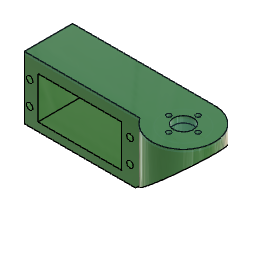
Coxa v8 (Autodesk Fusion 360 design; units mm, degrees)
Autodesk Fusion 360 part; units mm, degrees
sketch "Sketch1" plane through (0, 0, 0) normal (0, 0, 1) x (1, 0, 0)
  circle A0 centre (0, 0) radius 10
  dimension "d1" = 20
  constraint coincident A0.centre origin
  measures "d1" diameter of A0
extrude "Extrude1" add sketch "Sketch1" along normal blind 0.5 makes body 1
sketch "Sketch2" plane through (0, 0, 0) normal (0, 0, -1) x (1, 0, 0)
  circle A0 centre (0, 0) radius 10
  circle A1 centre (0, 0) radius 15
  dimension "d4" = 30
  constraint concentric A0 A1
  measures "d4" diameter of A1
extrude "Extrude2" add sketch "Sketch2" along normal blind 4 separate body makes body 2
sketch "Sketch3" plane through (0, 0, 0) normal (0, 1, 0) x (1, 0, 0)
sketch "Sketch4" plane through (0, 0, 0) normal (0, 1, 0) x (1, 0, 0)
  line L0 (-12.3324, 0) -> (-15, 0)
  line L1 (-12.3324, 3.9554) -> (-12.3324, 0)
  line L2 (-15.0407, 3.9554) -> (-47.0433, 16.0142)
  line L3 (-15, 0) -> (-47.0492, -12.0611)
  line L4 (-15.0407, 3.9554) -> (-12.3324, 3.9554)
  arc A0 (-47.0433, 16.0142) -> (-47.0492, -12.0611) centre (-52.3324, 1.9777) ccw
  dimension "d8" = 30
  constraint horizontal L0
  constraint vertical L1
  constraint tangent L2 A0
  constraint tangent L3 A0
  measures "d8" diameter of A0
extrude "Extrude3" add sketch "Sketch4" along normal mid plane 30 bodies 2
sketch "Sketch5" plane through (0, 0, 0) normal (0, 0, 1) x (1, 0, 0)
  line L0 (-12.2989, -8.5565) -> (-47, -8.5565)
  line L1 (-47, -8.5565) -> (-47, -15)
  line L2 (-47, -15) -> (-12.2989, -15)
  line L3 (-12.2989, -15) -> (-12.2989, -8.5565)
  line L4 (0, 15) -> (-13, 4.1667)
  line L5 (-13, 4.1667) -> (-13, 15)
  line L6 (-13, 15) -> (0, 15)
  line L7 (-13, 15) -> (-13.6576, 15)
  constraint horizontal L0
  constraint vertical L1
  constraint horizontal L2
  constraint vertical L3
  constraint vertical L5
  constraint perpendicular L5 L6
extrude "Extrude4" add sketch "Sketch5" against normal blind 4 contours L4 L5 L6 bodies 2
sketch "Sketch6" plane through (0, 0, 0) normal (0, 0, 1) x (1, 0, 0)
  line L0 (-12.3799, -8.5625) -> (-69, -8.5625)
  line L1 (-69, -8.5625) -> (-69, -16)
  line L2 (-69, -16) -> (-12.3799, -16)
  line L3 (-12.3799, -16) -> (-12.3799, -8.5625)
  constraint horizontal L0
  constraint vertical L1
  constraint horizontal L2
  constraint vertical L3
extrude "Extrude5" cut sketch "Sketch6" along normal mid plane 36 bodies 2
sketch "Sketch7" plane through (0, 0, 0) normal (0, 0, 1) x (1, 0, 0)
  line L0 (-12.38, -8.56) -> (-12.3324, -8.5389)
  line L1 (-12.3324, -8.5389) -> (-12.31, -15)
  line L2 (-12.31, -15) -> (-12.4048, -15.0003)
  line L3 (-12.4048, -15.0003) -> (-12.38, -8.56)
  constraint perpendicular L1 L2
extrude "Extrude6" cut 1 faces at (-12.3324, -10.6926, -1.3185) along direction (-1, 0, 0) blind 0.047 on bodies 2 bodies 2
extrude "Extrude7" cut sketch "Sketch7" against normal blind 4 bodies 2
sketch "Sketch8" plane through (0, 0, 0) normal (0, 1, 0) x (1, 0, 0)
  line L0 (-21.5442, 4.9968) -> (-61.5442, 4.9968)
  line L1 (-61.5442, 4.9968) -> (-61.5442, 25)
  line L2 (-61.5442, 25) -> (-21.5442, 25)
  line L3 (-21.5442, 25) -> (-21.5442, 4.9968)
  line L4 (-15, 0) -> (-67, 0)
  line L5 (-67, 0) -> (-67, 29)
  line L6 (-67, 29) -> (-15, 29)
  line L7 (-15, 29) -> (-15, 0)
  dimension "d19" = 40
  constraint horizontal L0
  constraint vertical L1
  constraint horizontal L2
  constraint vertical L3
  constraint horizontal L4
  constraint vertical L5
  constraint horizontal L6
  constraint vertical L7
  measures "d19" distance of L0.start L0.end
extrude "Extrude8" add sketch "Sketch8" along normal blind 15.01 and the other way blind -15 bodies 2
sketch "Sketch9" plane through (0, 15, 0) normal (0, 1, 0) x (-1, 0, 0)
  line L0 (21.5442, -4.9968) -> (21.5442, -6.4059)
  line L1 (21.5442, -6.4059) -> (47.0433, -16.0142)
  arc A0 (47.0433, -16.0142) -> (61.5442, -13.8158) centre (52.3324, -1.9777) ccw
  line L2 (61.5442, -13.8158) -> (61.5442, -4.9968)
  line L3 (61.5442, -4.9968) -> (21.5442, -4.9968)
  line L4 (61.5736, -19.9647) -> (21.5442, -19.9647)
  line L5 (21.5442, -19.9647) -> (21.5442, -4.9968)
  line L6 (21.5442, -4.9968) -> (61.5736, -4.9968)
  line L7 (61.5736, -4.9968) -> (61.5736, -19.9647)
  constraint horizontal L4
  constraint vertical L5
  constraint horizontal L6
  constraint vertical L7
  constraint coincident L0.start L3.end
extrude "Extrude9" cut sketch "Sketch9" against normal blind 27 contours L0 L1 A0 L2 L3 L5 L6 bodies 2
extrude "Extrude10" add 1 faces at (-17.1814, 15, -19.3185) along direction (0, -1, 0) blind 23 on bodies 2 bodies 2
extrude "Extrude11" cut 1 faces at (-43.0164, 15, 4.0204) along direction (0, -1, 0) blind 43 on bodies 2 bodies 2
sketch "Sketch10" plane through (0, 15.01, 0) normal (0, 1, 0) x (-1, 0, 0)
  line L0 (61.5442, -25) -> (21.5442, -25)
  line L1 (21.5442, -25) -> (21.5442, -4.9968)
  line L2 (21.5442, -4.9968) -> (61.5442, -4.9968)
  line L3 (61.5442, -4.9968) -> (61.5442, -25)
  line L4 (15, -29) -> (67, -29)
  line L5 (67, -29) -> (67, 0)
  line L6 (67, 0) -> (15, 0)
  line L7 (15, 0) -> (15, -29)
  line L8 (61.5442, -25) -> (21.5442, -25)
  line L9 (21.5442, -25) -> (21.5442, -4.9968)
  line L10 (21.5442, -4.9968) -> (61.5442, -4.9968)
  line L11 (61.5442, -4.9968) -> (61.5442, -25)
  line L12 (40, -14.9984) -> (40, -15.5643)
  line L13 (21.5442, -20.5643) -> (17.5442, -20.5643)
  circle A0 centre (17.5442, -20.5643) radius 1.5354
  circle A1 centre (17.5442, -9.4325) radius 1.5354
  line L14 (61.5442, -20.5643) -> (65.5, -20.5643)
  circle A2 centre (65.5, -20.5643) radius 0.9824
  circle A3 centre (65.5, -9.4325) radius 0.9824
  dimension "d31" = 4
  constraint horizontal L8
  constraint vertical L9
  constraint horizontal L10
  constraint vertical L11
  constraint coincident L1.end L2.start
  constraint coincident L0.start L3.end
  constraint coincident L1 L13.start
  constraint perpendicular L1 L13
  constraint coincident L13.end A0.centre
  constraint coincident L3 L14.start
  constraint perpendicular L3 L14
  constraint coincident L14.end A2.centre
  measures "d31" distance of L13.start L13.end
extrude "Extrude12" cut sketch "Sketch10" against normal blind 26 contours A0 | A1 | A2 | A3 bodies 2
extrude "Extrude13" add 1 faces at (2.0783, 2.6061, 0) along direction (0, 0, -1) blind 2 on bodies 1 bodies 1 2
sketch "Sketch11" plane through (-15, 0, 0) normal (1, 0, 0) x (0, 1, 0)
  line L0 (15, 0) -> (15, -3.9554)
  line L1 (15, -3.9554) -> (0, -3.9554)
  line L2 (0, -3.9554) -> (0, -4)
  line L3 (0, -4) -> (0, -3.9554)
  line L4 (0, -3.9554) -> (-8, -3.9554)
  line L5 (-8, -3.9554) -> (-8, -29)
  line L6 (-8, -29) -> (15.01, -29)
  line L7 (15.01, -29) -> (15.01, 0)
  line L8 (15.01, 0) -> (15, 0)
  line L9 (15, -3.9554) -> (-8, -3.9554)
  line L10 (-8, -3.9554) -> (-8, -29)
  line L11 (-8, -29) -> (15, -29)
  line L12 (15, -29) -> (15, -3.9554)
  constraint horizontal L9
  constraint vertical L10
  constraint horizontal L11
  constraint vertical L12
  constraint coincident L5.end L6.start
  constraint coincident L0.end L1.start
extrude "Extrude14" add sketch "Sketch11" along normal blind 30 contours L1 L4 L5 L6 L9 L10 L11 L12 bodies 1
sketch "Sketch12" plane through (0, 15, 0) normal (0, 1, 0) x (-1, 0, 0)
  line L0 (15, -29) -> (15, 0)
  line L1 (15, 0) -> (0, 0)
  line L2 (0, 0) -> (0, -3.9554)
  line L3 (0, -3.9554) -> (-15, -3.9554)
  line L4 (-15, -3.9554) -> (-15, -29)
  line L5 (-15, -29) -> (15, -29)
  line L6 (15, -29) -> (15, -28.4544)
  line L7 (-15, -3.9554) -> (15, -29)
  line L8 (-15, -29) -> (15, -29)
  line L9 (-15, -29) -> (-15, -3.9554)
  constraint coincident L0.start L5.end
  constraint coincident L0 L6.end
  constraint parallel L0 L6
  constraint coincident L3.end L4.start
  constraint coincident L4.end L5.start
extrude "Extrude15" cut sketch "Sketch12" against normal blind 26 contours L4 L5 L7 L8 L9 bodies 1
sketch "Sketch13" plane through (0, 0, -4) normal (0, 0, -1) x (1, 0, 0)
  line L0 (-12.6886, 8) -> (-6, 8)
  arc A0 (6, 8) -> (-6, 8) centre (0, 0) ccw
  line L1 (6, 8) -> (12.6886, 8)
  arc A1 (12.6886, 8) -> (-12.6886, 8) centre (0, 0) ccw
  circle A2 centre (0, 0) radius 10
  constraint concentric A0 A2
extrude "Extrude16" cut sketch "Sketch13" along normal blind 23 contours A0 A2 bodies 1
extrude "Extrude17" cut 1 faces at (0.857, -1.7143, -4) along direction (0, 0, 1) blind 3 on bodies 1 bodies 1
sketch "Sketch14" plane through (0, 0, 0) normal (0, 0, 1) x (-1, 0, 0)
  circle A0 centre (0, 0) radius 10
  line L0 (15, -15) -> (15, -15.01)
  line L1 (15, -15.01) -> (67, -15.01)
  line L2 (67, -15.01) -> (67, 8.5625)
  line L3 (67, 8.5625) -> (12.38, 8.5625)
  line L4 (12.38, 8.5625) -> (12.38, 8.56)
  line L5 (12.38, 8.56) -> (12.3794, 8.5597)
  line L6 (12.3794, 8.5597) -> (12.3794, 8.5388)
  line L7 (12.3794, 8.5388) -> (12.3324, 8.5388)
  arc A1 (12.3324, 8.5388) -> (0, -15) centre (0, 0) ccw
  line L8 (0, -15) -> (15, -15)
  line L9 (-12.669, 8.0309) -> (-15, 8.0309)
  line L10 (-15, 8.0309) -> (-15, -15)
  line L11 (-15, -15) -> (0, -15)
  arc A2 (-12.669, 8.0309) -> (0, -15) centre (0, 0) ccw
  constraint coincident A0.centre A1.centre
  constraint coincident A1 L9.start
  constraint horizontal L9
  constraint perpendicular L9 L10
  constraint coincident A1.end L8.start
  constraint tangent A1 L11
extrude "Extrude18" cut sketch "Sketch14" against normal blind 22 contours A1 L10 L11 A2 | A1 L9 L10 A2 bodies 1
extrude "Extrude19" add 1 faces at (0.9558, -13.273, -4) along direction (0, 0, -1) blind 24 on bodies 1 bodies 1
extrude "Extrude20" cut 1 faces at (-1.5996, -8.2578, -2) along direction (0, 0, 1) blind 1 on bodies 1 bodies 1
sketch "Sketch15" plane through (0, 15, 0) normal (0, 1, 0) x (-1, 0, 0)
  line L0 (0, -3.9554) -> (0, -16.4777)
  line L1 (0, -16.4777) -> (15, -29)
  line L2 (15, -29) -> (15, 0)
  line L3 (15, 0) -> (0, 0)
  line L4 (0, 0) -> (0, -3.9554)
  line L5 (15, -29) -> (-15.1205, -3.8547)
  line L6 (-15.1205, -3.8547) -> (-15.1205, -28)
  line L7 (-15.1205, -28) -> (15, -29)
  constraint coincident L1.end L2.start
  constraint parallel L1 L5
  constraint parallel L2 L6
extrude "Extrude21" cut sketch "Sketch15" against normal blind 43 contours L1 L5 L6 L7 bodies 1
sketch "Sketch16" plane through (0, 0, -1) normal (0, 0, -1) x (1, 0, 0)
  circle A0 centre (0, 0) radius 10
  circle A1 centre (0, 0) radius 2.5
  line L0 (0, 0) -> (7, 0)
  circle A2 centre (7, 0) radius 1.5
  line L1 (0, 0) -> (0, 7)
  circle A3 centre (0, 7) radius 1.5
  line L2 (0, 0) -> (0, -7)
  circle A4 centre (7, 0) radius 1.5
  circle A5 centre (0, -7) radius 1.5
  line L3 (0, 0) -> (-7, 0)
  circle A6 centre (-7, 0) radius 1.5
  dimension "d52" = 5
  dimension "d53" = 7
  dimension "d54" = 3
  dimension "d55" = 7
  dimension "d56" = 3
  dimension "d57" = 7
  dimension "d58" = 3
  dimension "d59" = 3
  dimension "d60" = 7
  dimension "d61" = 3
  constraint coincident A0.centre A1.centre
  constraint horizontal L0
  constraint coincident L0.end A2.centre
  constraint perpendicular L0 L1
  constraint coincident L1.end A3.centre
  constraint perpendicular L0 L2
  constraint coincident L2.end A5.centre
  constraint perpendicular L1 L3
  constraint coincident L3.end A6.centre
  measures "d52" diameter of A1
  measures "d53" distance of A0.centre L0.end
  measures "d54" diameter of A2
  measures "d55" distance of A0.centre L1.end
  measures "d56" diameter of A3
  measures "d57" distance of A0.centre L2.end
  measures "d58" diameter of A4
  measures "d59" diameter of A5
  measures "d60" distance of A0.centre L3.end
  measures "d61" diameter of A6
extrude "Extrude22" cut sketch "Sketch16" against normal blind 4 contours A1 L0 L1 | A1 L0 L2 | A1 L1 L3 | A1 L2 L3 | A2 A4 | A3 | A5 | A6 bodies 1
sketch "Sketch17" plane through (0, 0, 0.5) normal (0, 0, 1) x (-1, 0, 0)
  circle A0 centre (-7, 0) radius 1.5
  circle A1 centre (0, 0) radius 2.5
  circle A2 centre (0, -7) radius 1.5
  circle A3 centre (0, 7) radius 1.5
  circle A4 centre (7, 0) radius 1.5
  circle A5 centre (0, 0) radius 10
  circle A6 centre (0, 0) radius 4
  circle A7 centre (0, 0) radius 11
  dimension "d64" = 8
  dimension "d65" = 22
  constraint coincident A1.centre A5.centre
  constraint concentric A6 A7
  measures "d64" diameter of A6
  measures "d65" diameter of A7
extrude "Extrude23" cut sketch "Sketch17" against normal blind 13 contours A6 bodies 1
sketch "Sketch18" plane through (0, 0, -1) normal (0, 0, -1) x (1, 0, 0)
  circle A0 centre (0, 0) radius 4
  circle A1 centre (7, 0) radius 1.5
  circle A2 centre (0, -7) radius 1.5
  circle A3 centre (0, 7) radius 1.5
  circle A4 centre (-7, 0) radius 1.5
  circle A5 centre (0, 0) radius 10
  circle A6 centre (0, 0) radius 11
  dimension "d68" = 22
  constraint coincident A0.centre A5.centre
  measures "d68" diameter of A6
extrude "Extrude24" cut sketch "Sketch18" along normal blind 26 contours A6 bodies 1
sketch "Sketch19" plane through (0, 0, -29) normal (0, 0, -1) x (1, 0, 0)
  line L0 (-15, -15) -> (-15, 8)
  line L1 (-15, 8) -> (-67, 8)
  line L2 (-67, 8) -> (-67, -15.01)
  line L3 (-67, -15.01) -> (-15, -15.01)
  line L4 (-15, -15.01) -> (-15, -15)
  line L5 (-15, 8) -> (-67, 8)
  line L6 (-67, 8) -> (-67, 12)
  line L7 (-67, 12) -> (-67, 13)
  line L8 (-67, 13) -> (-67, 12)
  line L9 (-15, 8) -> (-15, 13)
  line L10 (-15, 13) -> (-15, 14)
  line L11 (-15, 14) -> (-67, 13)
  constraint coincident L0.end L1.start
  constraint coincident L1.end L2.start
  constraint perpendicular L5 L6
  constraint perpendicular L5 L7
  constraint perpendicular L1 L8
  constraint perpendicular L5 L9
  constraint perpendicular L5 L10
extrude "Extrude25" cut sketch "Sketch19" against normal blind 30 contours L1 L5 L6 L7 L8 L9 L10 L11 bodies 1
sketch "Sketch20" plane through (0, 0, -29) normal (0, 0, -1) x (1, 0, 0)
  line L0 (-15, -15) -> (-15, 8)
  line L1 (-15, 8) -> (-67, 8)
  line L2 (-67, 8) -> (-67, -15.01)
  line L3 (-67, -15.01) -> (-15, -15.01)
  line L4 (-15, -15.01) -> (-15, -15)
  spline S0 degree 5 poles (-12.3276, 8.5412) (-12.3307, 8.538) (-12.3371, 8.5312) (-12.3476, 8.5193) (-12.3632, 8.5002) (-12.3854, 8.471) (-12.4103, 8.4364) (-12.4378, 8.3967) (-12.4673, 8.3527) (-12.4982, 8.3058) (-12.5295, 8.2576) (-12.5604, 8.2099) (-12.5899, 8.1644) (-12.6173, 8.1223) (-12.6422, 8.0845) (-12.6644, 8.0513) (-12.68, 8.0285) (-12.6904, 8.0134) (-12.6969, 8.0043) (-12.7, 8) knots 0 0 0 0 0 0 0.066667 0.133333 0.2 0.266667 0.333333 0.4 0.466667 0.533333 0.6 0.666667 0.733333 0.8 0.866667 0.933333 1 1 1 1 1 1
  line L5 (-12.7, 8) -> (-15, 8)
  line L6 (-15, 8.5635) -> (-12.3276, 8.6006)
  line L7 (-12.3276, 8.6006) -> (-12.3276, 8.5412)
  line L8 (-15, 8.5635) -> (-15, 8)
  line L9 (-15, 8.5635) -> (-12.7, 8.5635)
  line L10 (-12.7, 8.5635) -> (-12.7, 8)
  line L11 (-12.7, 8) -> (-15, 8)
  line L12 (-15, 8) -> (-15, 8.5635)
  point P0 (-12.4352, 8.4002)
  point P1 (-12.5911, 8.1626)
  constraint coincident L0.end L1.start
  constraint vertical L7
  constraint parallel L0 L8
  constraint horizontal L9
  constraint vertical L10
  constraint horizontal L11
  constraint vertical L12
extrude "Extrude26" cut sketch "Sketch20" against normal blind 35 contours L5 L8 L9 L10 L11 L12 | S0 L6 L7 L9 L10 bodies 1
delete_face "DeleteFace1" 2 faces at (-12.4882, -8.3094, -11.5883) (-12.6545, -8.0591, -3.9554) on bodies 1
move_face "OffsetFaces1" offset 1 1 faces at (-67, -0.33, -19.3333) on bodies 1
sketch "Sketch21" plane through (0, 15.01, 0) normal (0, 1, 0) x (-1, 0, 0)
  circle A0 centre (17.5442, -9.4325) radius 1.5354
  circle A1 centre (65.5, -9.4325) radius 0.9824
  circle A2 centre (17.5442, -20.5643) radius 1.5354
  circle A3 centre (65.5, -20.5643) radius 0.9824
  line L0 (61.5442, -25) -> (21.5442, -25)
  line L1 (21.5442, -25) -> (21.5442, -4.9968)
  line L2 (21.5442, -4.9968) -> (61.5442, -4.9968)
  line L3 (61.5442, -4.9968) -> (61.5442, -25)
  line L4 (15, -29) -> (68, -29)
  line L5 (68, -29) -> (68, 0)
  line L6 (68, 0) -> (15, 0)
  line L7 (15, 0) -> (15, -29)
  circle A4 centre (65.5, -20.5643) radius 1.5
  circle A5 centre (65.5, -9.4325) radius 1.5
  dimension "d76" = 3
  dimension "d77" = 3
  constraint concentric A3 A4
  constraint concentric A1 A5
  measures "d76" diameter of A4
  measures "d77" diameter of A5
extrude "Extrude27" cut sketch "Sketch21" against normal blind 24 contours A4 | A5 bodies 1
sketch "Sketch22" plane through (0, 0, 0) normal (0, 0, 1) x (-1, 0, 0)
  line L0 (12.3276, 8.5412) -> (12.3276, 8.5458)
  arc A0 (12.3276, 8.5458) -> (0, -15) centre (0, 0) ccw
  line L1 (0, -15) -> (15, -15)
  line L2 (15, -15) -> (15, -15.01)
  line L3 (15, -15.01) -> (68, -15.01)
  line L4 (68, -15.01) -> (68, 8)
  line L5 (68, 8) -> (12.7, 8)
  spline S0 degree 3 poles (12.7, 8) (12.6517, 8.0675) (12.5788, 8.182) (12.4451, 8.3873) (12.3732, 8.4946) (12.3276, 8.5412) knots 0 0 0 0 0.024897 0.024897 0.051258 0.051258 0.051258 0.051258
  circle A1 centre (0, 0) radius 10
extrude "Extrude28" add 1 faces at (-50.3333, 7.3367, 0) along direction (0, 0, 1) blind 0.5 on bodies 1 bodies 1
move_face "OffsetFaces2" offset 1 1 faces at (-5.8986, 3.7831, -1) on bodies 1
sketch "Sketch23" plane through (0, 0, -2) normal (0, 0, -1) x (1, 0, 0)
  circle A0 centre (0, 0) radius 11
  circle A1 centre (0, 0) radius 4
  circle A2 centre (7, 0) radius 1.5
  circle A3 centre (0, -7) radius 1.5
  circle A4 centre (0, 7) radius 1.5
  circle A5 centre (-7, 0) radius 1.5
  circle A6 centre (0, 0) radius 4.75
  dimension "d83" = 9.5
  constraint coincident A0.centre A1.centre
  measures "d83" diameter of A6
extrude "Extrude29" cut sketch "Sketch23" against normal blind 5 contours A6 bodies 1
sketch "Sketch24" plane through (0, 0, -2) normal (0, 0, -1) x (1, 0, 0)
  circle A0 centre (0, 0) radius 4.75
  circle A1 centre (0, 0) radius 11
  circle A2 centre (7, 0) radius 1.5
  circle A3 centre (0, -7) radius 1.5
  circle A4 centre (0, 7) radius 1.5
  circle A5 centre (-7, 0) radius 1.5
  circle A6 centre (0, -7) radius 1.118
  circle A7 centre (0, -7) radius 1.5
  circle A8 centre (7, 0) radius 1.118
  circle A9 centre (7, 0) radius 1.5
  circle A10 centre (0, 7) radius 1.118
  circle A11 centre (0, 7) radius 1.5
  circle A12 centre (-7, 0) radius 1.118
  circle A13 centre (-7, 0) radius 1.5
  dimension "d87" = 360
  constraint concentric A3 A6
  constraint concentric A6 A7
extrude "Extrude30" add sketch "Sketch24" against normal blind 2.5 contours A2 A9 | A3 A7 | A4 A11 | A5 A13 bodies 1
sketch "Sketch25" plane through (0, 0, 0) normal (0, 0, 1) x (-1, 0, 0)
move_face "OffsetFaces3" offset 1 1 faces at (-50.3333, 7.3367, 0.5) on bodies 1
sketch "Sketch26" plane through (0, 0, 0) normal (0, 1, 0) x (1, 0, 0)
move_face "OffsetFaces4" offset -0.5 1 faces at (-50.3333, 7.3367, 1.5) on bodies 1
sketch "Sketch27" plane through (0, 0, 1) normal (0, 0, 1) x (-1, 0, 0)
  circle A0 centre (7, 0) radius 1.118
  circle A1 centre (0, -7) radius 1.118
  circle A2 centre (0, 7) radius 1.118
  circle A3 centre (-7, 0) radius 1.118
  circle A4 centre (0, 0) radius 4.75
  line L0 (12.3276, 8.5412) -> (12.3276, 8.5458)
  arc A5 (12.3276, 8.5458) -> (0, -15) centre (0, 0) ccw
  line L1 (0, -15) -> (15, -15)
  line L2 (15, -15) -> (15, -15.01)
  line L3 (15, -15.01) -> (68, -15.01)
  line L4 (68, -15.01) -> (68, 8)
  line L5 (68, 8) -> (12.7, 8)
  spline S0 degree 3 poles (12.7, 8) (12.629, 8.0992) (12.5086, 8.295) (12.391, 8.4638) (12.3554, 8.5127) (12.3276, 8.5412) knots -0.04982 -0.04982 -0.04982 -0.04982 -0.011937 -0.011937 0 0 0 0
